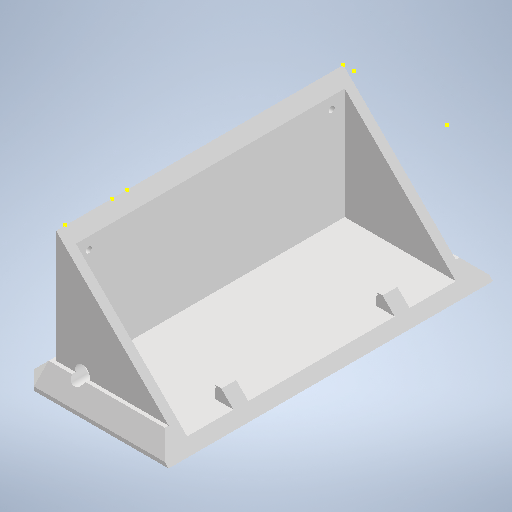
# Autodesk Inventor part: manuDisplayHolder
Saved by Autodesk Inventor 2025 (Build 290162000, 162)
## iProperties
Created: 2024-04-01
Part Number: manuDisplayHolder
Material: Generic
Document SubType Name: Modeling
Designer: 48791
Density: 1 g/cm^3
Appearance: Default
Author: 48791
Autodesk Inventor part; units mm, degrees
ref_plane "YZ Plane" through (0, 0, 0) normal (1, 0, 0) x (0, 1, 0)
ref_plane "XZ Plane" through (0, 0, 0) normal (0, 1, 0) x (-1, 0, 0)
sketch "Sketch1" plane through (0, 0, 0) normal (0, 0, 1) x (1, 0, 0)
  line L0 (0, 0) -> (0, -70.71)
  line L1 (0, -70.71) -> (70.71, -70.71)
  line L2 (70.71, -70.71) -> (0, 0)
  dimension "d0" = 70.71
  dimension "d1" = 70.71
  constraints: 6 end point, 1 perpendicular, 1 vertical
  measures "d0" distance of L0.start L0.end
  measures "d1" distance of L0.end L1.end
extrude "Extrusion1" add sketch "Sketch1" along normal blind 155
sketch "Sketch2" plane through (0, -70.71, 0) normal (0, -1, 0) x (1, 0, 0)
  point P0 (0, 0)
sketch "Sketch3" plane through (0, -70.71, 0) normal (0, -1, 0) x (1, 0, 0)
  point P0 (0, 0)
sketch "Sketch4" plane through (0, -70.71, 0) normal (0, -1, 0) x (1, 0, 0)
  point P0 (0, 0)
sketch "Sketch5" plane through (0, -70.71, 0) normal (0, -1, 0) x (1, 0, 0)
  line L0 (65.71, 150) -> (5.71, 150)
  line L1 (5.71, 150) -> (5.71, 5)
  line L2 (5.71, 5) -> (65.71, 5)
  line L3 (65.71, 5) -> (65.71, 150)
  line L4 (70.71, 0) -> (70.71, 155) projected
  line L5 (0, 0) -> (70.71, 0) projected
  dimension "d4" = 60
  dimension "d5" = 145
  dimension "d6" = 5
  dimension "d7" = 5
  constraints: 8 end point, 2 parallel, 1 horizontal, 1 perpendicular
  measures "d4" distance of L2.end L1.end
  measures "d5" distance of L1.end L0.end
  measures "d6" distance between parallel lines of L4 L3
  measures "d7" distance between parallel lines of L5 L2
extrude "Extrusion2" cut sketch "Sketch5" against normal blind 155
sketch "Sketch6" plane through (5.71, -70.71, 150) normal (1, 0, 0) x (0, 0, -1)
  line L0 (0, 0) -> (145, 0)
  line L1 (145, 0) -> (145, 5)
  line L2 (145, 5) -> (0, 5)
  line L3 (0, 5) -> (0, 0)
  point P0 (150, 70.71)
  dimension "d10" = 145
  dimension "d11" = 5
  constraints: 8 end point, 2 parallel, 1 horizontal, 1 perpendicular
  measures "d10" distance of L2.end L1.end
  measures "d11" distance of L1.end L0.end
extrude "Extrusion3" add sketch "Sketch6" along normal blind 60
sketch "Sketch7" plane through (5.71, -5.71, 150) normal (1, 0, 0) x (0, 0, -1)
  point P0 (150, 5.71)
sketch "Sketch8" plane through (65.71, -65.71, 150) normal (0, 0, -1) x (-1, 0, 0)
  point P0 (65.71, 65.71)
sketch "Sketch9" plane through (5.71, -65.71, 150) normal (0, 1, 0) x (1, 0, 0)
  point P0 (-5.71, 150)
sketch "Sketch10" plane through (5.71, -65.71, 150) normal (0, 1, 0) x (1, 0, 0)
  line L0 (60, 145) -> (60, 0) projected
  line L1 (60, 25) -> (50, 25)
  line L2 (50, 25) -> (50, 33)
  line L3 (50, 33) -> (60, 33)
  line L4 (60, 33) -> (60, 25)
  line L5 (60, 112) -> (50, 112)
  line L6 (50, 112) -> (50, 120)
  line L7 (50, 120) -> (60, 120)
  line L8 (60, 120) -> (60, 112)
  line L9 (60, 0) -> (0, 0) projected
  line L10 (0, 145) -> (60, 145) projected
  point P0 (-5.71, 150)
  point P1 (55, 25)
  point P2 (55, 120)
  point P3 (60, 33)
  dimension "d14" = 10
  dimension "d15" = 8
  dimension "d16" = 10
  dimension "d17" = 8
  dimension "d18" = 25
  dimension "d19" = 25
  constraints: 16 end point, 4 parallel, 2 horizontal, 2 midpoint, 2 perpendicular, 2 point on line
  measures "d14" distance of L2.end L3.end
  measures "d15" distance of L1.end L2.end
  measures "d16" distance of L6.end L7.end
  measures "d17" distance of L5.end L6.end
  measures "d18" distance from line of L9 point (55, 25)
  measures "d19" distance from line of L10 point (55, 120)
extrude "Extrusion4" add sketch "Sketch10" along normal blind 10
sketch "Sketch11" plane through (65.71, -65.71, 117) normal (0, 0, -1) x (-1, 0, 0)
  point P0 (65.71, 65.71)
sketch "Sketch12" plane through (65.71, -65.71, 117) normal (0, 0, -1) x (-1, 0, 0)
  line L0 (0, 10) -> (10, 10) projected
  line L1 (0, 0) -> (0, 10)
  line L2 (0, 10) -> (10, 10)
  line L3 (10, 10) -> (0, 0)
  point P0 (65.71, 65.71)
  constraints: 6 end point, 2 perpendicular
extrude "Extrusion5" cut sketch "Sketch12" against normal blind 15
sketch "Sketch13" plane through (65.71, -65.71, 30) normal (0, 0, -1) x (-1, 0, 0)
  line L0 (0, 0) -> (10, 0) projected
  line L1 (0, 0) -> (0, 10) projected
  line L2 (0, 0) -> (0, 10)
  line L3 (10, 0) -> (10, 10) projected
  line L4 (0, 10) -> (10, 10)
  line L5 (10, 10) -> (0, 0)
  point P0 (65.71, 65.71)
  constraints: 6 end point, 1 collinear, 1 perpendicular
extrude "Extrusion6" cut sketch "Sketch13" against normal blind 15 contours L1 L4 L5
sketch "Sketch14" plane through (65.71, -65.71, 150) normal (0, 0, -1) x (-1, 0, 0)
  circle A0 centre (51.4521, 6.4297) radius 4
  point P0 (65.71, 65.71)
  dimension "d26" = 8
  constraints: 1 centre point
  measures "d26" diameter of A0
extrude "Extrusion7" cut sketch "Sketch14" against normal blind 15
sketch "Sketch15" plane through (0, 0, 0) normal (0.7071068, 0.7071068, 0) x (-0.7071068, 0.7071068, 0)
  point P0 (0, 0)
sketch "Sketch16" plane through (0, 0, 0) normal (0.7071068, 0.7071068, 0) x (-0.7071068, 0.7071068, 0)
  point P0 (0, 0)
sketch "Sketch17" plane through (55.71, -65.71, 30) normal (-1, 0, 0) x (0, 0, 1)
  point P0 (-30, 65.71)
sketch "Sketch18" plane through (55.71, -65.71, 30) normal (-1, 0, 0) x (0, 0, 1)
  point P0 (-30, 65.71)
sketch "Sketch19" plane through (55.71, -65.71, 125) normal (0, 0, 1) x (1, 0, 0)
  point P0 (-55.71, 65.71)
sketch "Sketch20" plane through (55.71, -65.71, 125) normal (0, 0, 1) x (1, 0, 0)
  line L0 (-7.5736, 14.1421) -> (0.9117, 5.6569)
  line L1 (0.9117, 5.6569) -> (6.5685, 0)
  line L2 (6.5685, 0) -> (-0.5025, 0)
  line L3 (-0.5025, 0) -> (-2.6238, 2.1213)
  line L4 (-2.6238, 2.1213) -> (-4.0381, 3.5355)
  line L5 (-4.0381, 3.5355) -> (-2.2703, 5.3033)
  line L6 (-2.2703, 5.3033) -> (-9.3414, 12.3744)
  line L7 (-9.3414, 12.3744) -> (-7.5736, 14.1421)
  line L8 (0.9117, 5.6569) -> (-2.6238, 2.1213)
  line L9 (-46.4645, 45.9619) -> (-50, 49.4975)
  line L10 (-50, 49.4975) -> (-50, 56.5685)
  line L11 (-50, 56.5685) -> (-35.8579, 42.4264)
  line L12 (-35.8579, 42.4264) -> (-37.6256, 40.6586)
  line L13 (-37.6256, 40.6586) -> (-44.6967, 47.7297)
  line L14 (-44.6967, 47.7297) -> (-46.4645, 45.9619)
  point P0 (-55.71, 65.71)
  constraints: 30 end point, 1 horizontal, 1 vertical, 27 other
extrude "Extrusion8" cut sketch "Sketch20" against normal up to surface (95 mm away) contours L0 L8 L4 L5 L6 L7
sketch "Sketch21" plane through (0, -70.71, 0) normal (0, -1, 0) x (1, 0, 0)
  line L0 (0, 0) -> (70.71, 0) projected
  line L1 (70.71, 0) -> (70.71, 155) projected
  line L2 (0, 155) -> (70.71, 155) projected
  line L3 (0, 0) -> (0, 155) projected
  line L4 (-10, 165) -> (70.71, 165)
  line L5 (70.71, -10) -> (-10, -10)
  line L6 (-10, -10) -> (-10, 165)
  line L7 (0, 77.5) -> (70.71, 77.5)
  line L8 (35.355, 0) -> (35.355, 155)
  line L9 (70.71, 0) -> (70.71, 155) projected
  line L10 (70.71, -10) -> (70.71, 165)
  dimension "d31" = 10
  dimension "d32" = 10
  constraints: 12 end point, 4 midpoint, 2 point on line, 1 perpendicular, 1 other
  measures "d31" distance between parallel lines of L3 L6
  measures "d32" distance between parallel lines of L4 L2
extrude "Extrusion9" add sketch "Sketch21" against normal blind 10 contours L0 L10 L5 L6 L4 L2 L3
chamfer "Chamfer1" distance 8 angle 45 5 edges at (-10, -60.71, 77.5) (30.355, -60.71, 165) (-10, -65.71, 165) (30.355, -60.71, -10) (-10, -65.71, -10)
sketch "Sketch22" plane through (-2, -70.71, 165) normal (0, 0, 1) x (1, 0, 0)
  line L0 (72.71, 0) -> (62.71, 10) projected
  line L1 (72.71, 10) -> (62.71, 10) projected
  line L2 (72.71, 0) -> (72.71, 10) projected
  point P0 (2, 70.71)
extrude "Extrusion10" cut sketch "Sketch22" against normal blind 228.125
sketch "Sketch23" plane through (0, 0, 0) normal (-1, 0, 0) x (0, 0, 1)
  line L0 (36.1859, -20.6342) -> (112.0724, -20.6342) construction
  line L1 (112.0724, -20.6342) -> (112.0724, -41.0586) construction
  line L2 (112.0724, -41.0586) -> (36.1859, -41.0586) construction
  line L3 (36.1859, -41.0586) -> (36.1859, -20.6342) construction
  line L4 (0, -60.71) -> (155, -60.71) projected
  line L5 (155, 0) -> (155, -60.71) projected
  line L6 (0, 0) -> (155, 0) projected
  line L7 (0, 0) -> (0, -60.71) projected
  line L8 (0, 0) -> (155, 0) projected
  line L9 (74.1291, 0) -> (74.1291, -60.71) construction
  spline S0 degree 2 poles (50.979, -23.8756) (50.7548, -23.8756) (49.6859, -23.6859) (49.3928, -23.6859) knots 0 0 0 1 2 2 2
  spline S1 degree 2 poles (49.3928, -23.6859) (48.7893, -23.6859) (47.9617, -23.7204) knots 0 0 0 1 1 1
  line L10 (47.9617, -23.7204) -> (48.0307, -25.1859)
  spline S2 degree 2 poles (48.0307, -25.1859) (48.0307, -34.3928) (46.8066, -38.5825) knots 0 0 0 1 1 1
  spline S3 degree 2 poles (46.8066, -38.5825) (45.9962, -41.3583) (43.9445, -41.3583) knots 0 0 0 1 1 1
  spline S4 degree 2 poles (43.9445, -41.3583) (41.7893, -41.3583) (39.6859, -39.8066) knots 0 0 0 1 1 1
  spline S5 degree 2 poles (39.6859, -39.8066) (37.341, -38.0652) (37.341, -35.8238) knots 0 0 0 1 1 1
  spline S6 degree 2 poles (37.341, -35.8238) (37.341, -34.3066) (38.5997, -34.3066) knots 0 0 0 1 1 1
  spline S7 degree 2 poles (38.5997, -34.3066) (39.841, -34.3066) (39.841, -35.8066) knots 0 0 0 1 1 1
  spline S8 degree 2 poles (39.841, -35.8066) (39.841, -36.8238) (41.3066, -37.8411) knots 0 0 0 1 1 1
  spline S9 degree 2 poles (41.3066, -37.8411) (42.7031, -38.8066) (43.9445, -38.8066) knots 0 0 0 1 1 1
  spline S10 degree 2 poles (43.9445, -38.8066) (44.9617, -38.8066) (45.3583, -32.5825) knots 0 0 0 1 1 1
  spline S11 degree 2 poles (45.3583, -32.5825) (45.5479, -29.6514) (45.5479, -25.1859) knots 0 0 0 1 1 1
  spline S12 degree 2 poles (45.5479, -25.1859) (45.5479, -24.8411) (45.479, -23.8583) knots 0 0 0 1 1 1
  line L11 (45.479, -23.8583) -> (44.7376, -23.8756)
  spline S13 degree 2 poles (44.7376, -23.8756) (44.2548, -23.8756) (42.3066, -23.8066) (41.8238, -23.8066) knots 0 0 0 1 2 2 2
  spline S14 degree 2 poles (41.8238, -23.8066) (41.2721, -23.8066) (40.5307, -23.117) (40.5307, -22.5135) knots 0 0 0 1 2 2 2
  spline S15 degree 2 poles (40.5307, -22.5135) (40.5307, -21.2376) (42.2548, -21.2376) knots 0 0 0 1 1 1
  spline S16 degree 2 poles (42.2548, -21.2376) (42.6686, -21.2376) (44.3238, -21.3238) (44.7376, -21.3238) knots 0 0 0 1 2 2 2
  spline S17 degree 2 poles (44.7376, -21.3238) (45.5135, -21.3238) (48.6169, -21.1342) (49.3928, -21.1342) knots 0 0 0 1 2 2 2
  spline S18 degree 2 poles (49.3928, -21.1342) (52.2031, -21.1342) (52.2031, -22.5652) knots 0 0 0 1 1 1
  spline S19 degree 2 poles (52.2031, -22.5652) (52.2031, -23.0652) (51.8755, -23.4445) knots 0 0 0 1 1 1
  spline S20 degree 2 poles (51.8755, -23.4445) (51.5135, -23.8756) (50.979, -23.8756) knots 0 0 0 1 1 1
  spline S21 degree 2 poles (64.2893, -32.2894) (64.979, -32.7894) (65.9962, -33.8583) knots 0 0 0 1 1 1
  spline S22 degree 2 poles (65.9962, -33.8583) (67.1859, -35.0997) (68.0824, -35.8756) (68.0824, -36.3238) knots 0 0 0 1 2 2 2
  spline S23 degree 2 poles (68.0824, -36.3238) (68.0824, -36.7894) (67.41, -37.479) (66.979, -37.479) knots 0 0 0 1 2 2 2
  spline S24 degree 2 poles (66.979, -37.479) (66.6169, -37.479) (66.2721, -37.2204) knots 0 0 0 1 1 1
  spline S25 degree 2 poles (66.2721, -37.2204) (65.7893, -36.8583) (64.1686, -35.1687) knots 0 0 0 1 1 1
  spline S26 degree 2 poles (64.1686, -35.1687) (62.9272, -33.8756) (61.7721, -33.4273) knots 0 0 0 1 1 1
  spline S27 degree 2 poles (61.7721, -33.4273) (60.841, -33.0825) (60.841, -32.3928) knots 0 0 0 1 1 1
  spline S28 degree 2 poles (60.841, -32.3928) (60.841, -31.7721) (61.6859, -31.3756) knots 0 0 0 1 1 1
  spline S29 degree 2 poles (61.6859, -31.3756) (62.841, -30.8066) (64.2204, -29.3583) knots 0 0 0 1 1 1
  spline S30 degree 2 poles (64.2204, -29.3583) (66.1341, -27.3583) (66.8583, -26.7549) (67.2376, -26.7549) knots 0 0 0 1 2 2 2
  spline S31 degree 2 poles (67.2376, -26.7549) (67.6859, -26.7549) (68.3583, -27.4273) (68.3583, -27.8928) knots 0 0 0 1 2 2 2
  spline S32 degree 2 poles (68.3583, -27.8928) (68.3583, -28.3066) (67.979, -28.6859) knots 0 0 0 1 1 1
  spline S33 degree 2 poles (67.979, -28.6859) (66.8066, -29.9445) (64.2893, -32.2894) knots 0 0 0 1 1 1
  spline S34 degree 2 poles (77.7376, -40.4445) (75.8755, -40.4445) (74.3928, -39.6687) knots 0 0 0 1 1 1
  spline S35 degree 2 poles (74.3928, -39.6687) (72.7204, -38.7549) (72.1341, -37.1342) knots 0 0 0 1 1 1
  spline S36 degree 2 poles (72.1341, -37.1342) (72.0652, -36.9101) (72.0652, -36.7032) knots 0 0 0 1 1 1
  spline S37 degree 2 poles (72.0652, -36.7032) (72.0652, -36.2032) (72.8238, -35.548) (73.3238, -35.548) knots 0 0 0 1 2 2 2
  spline S38 degree 2 poles (73.3238, -35.548) (73.8066, -35.548) (74.1686, -35.9963) knots 0 0 0 1 1 1
  line L12 (74.1686, -35.9963) -> (74.7376, -36.8583)
  spline S39 degree 2 poles (74.7376, -36.8583) (75.1859, -37.4618) (76.6859, -38.0652) (77.7376, -38.0652) knots 0 0 0 1 2 2 2
  spline S40 degree 2 poles (77.7376, -38.0652) (79.0997, -38.0652) (80.1169, -37.2204) knots 0 0 0 1 1 1
  spline S41 degree 2 poles (80.1169, -37.2204) (81.1859, -36.3411) (81.1859, -35.048) knots 0 0 0 1 1 1
  spline S42 degree 2 poles (81.1859, -35.048) (81.1859, -33.1859) (79.8066, -32.0652) knots 0 0 0 1 1 1
  spline S43 degree 2 poles (79.8066, -32.0652) (78.5997, -31.0997) (76.5997, -30.8928) knots 0 0 0 1 1 1
  spline S44 degree 2 poles (76.5997, -30.8928) (75.2204, -30.7549) (75.2204, -29.7721) knots 0 0 0 1 1 1
  spline S45 degree 2 poles (75.2204, -29.7721) (75.2204, -29.048) (76.2893, -28.6687) knots 0 0 0 1 1 1
  line L13 (76.2893, -28.6687) -> (79.2548, -27.9445)
  spline S46 degree 2 poles (79.2548, -27.9445) (80.0997, -27.6342) (80.9617, -26.5825) (80.979, -25.8238) knots 0 0 0 1 2 2 2
  spline S47 degree 2 poles (80.979, -25.8238) (80.9962, -24.7376) (80.1341, -24.0652) knots 0 0 0 1 1 1
  spline S48 degree 2 poles (80.1341, -24.0652) (79.2376, -23.3756) (77.5997, -23.3756) knots 0 0 0 1 1 1
  spline S49 degree 2 poles (77.5997, -23.3756) (76.7548, -23.3756) (75.979, -23.7894) knots 0 0 0 1 1 1
  line L14 (75.979, -23.7894) -> (74.5824, -24.6687)
  spline S50 degree 2 poles (74.5824, -24.6687) (74.1686, -24.9273) (73.9272, -24.9273) knots 0 0 0 1 1 1
  spline S51 degree 2 poles (73.9272, -24.9273) (73.4272, -24.9273) (72.7204, -24.1687) (72.7204, -23.6859) knots 0 0 0 1 2 2 2
  spline S52 degree 2 poles (72.7204, -23.6859) (72.7204, -22.7032) (74.6169, -21.8066) knots 0 0 0 1 1 1
  spline S53 degree 2 poles (74.6169, -21.8066) (76.2548, -20.9963) (77.3238, -20.9963) knots 0 0 0 1 1 1
  spline S54 degree 2 poles (77.3238, -20.9963) (79.979, -20.9963) (81.5307, -22.1687) knots 0 0 0 1 1 1
  spline S55 degree 2 poles (81.5307, -22.1687) (83.2031, -23.4273) (83.2031, -25.7721) knots 0 0 0 1 1 1
  spline S56 degree 2 poles (83.2031, -25.7721) (83.2031, -28.6859) (80.8583, -29.5997) knots 0 0 0 1 1 1
  spline S57 degree 2 poles (80.8583, -29.5997) (80.6514, -29.6859) (80.3755, -29.7721) knots 0 0 0 1 1 1
  spline S58 degree 2 poles (80.3755, -29.7721) (82.0135, -30.3928) (83.6514, -32.8066) (83.6514, -34.5997) knots 0 0 0 1 2 2 2
  spline S59 degree 2 poles (83.6514, -34.5997) (83.6514, -37.048) (80.2204, -40.4445) (77.7376, -40.4445) knots 0 0 0 1 2 2 2
  spline S60 degree 2 poles (106.5997, -39.7894) (104.6859, -41.0997) (101.0824, -41.0997) knots 0 0 0 1 1 1
  spline S61 degree 2 poles (101.0824, -41.0997) (100.1859, -41.0997) (99.0307, -40.8066) knots 0 0 0 1 1 1
  spline S62 degree 2 poles (99.0307, -40.8066) (97.6341, -40.479) (96.9272, -39.9445) knots 0 0 0 1 1 1
  line L15 (96.9272, -39.9445) -> (96.7893, -39.9445)
  spline S63 degree 2 poles (96.7893, -39.9445) (96.2721, -39.9445) (95.5479, -39.2032) (95.5479, -38.6687) knots 0 0 0 1 2 2 2
  spline S64 degree 2 poles (95.5479, -38.6687) (95.5479, -37.3756) (95.7893, -32.2032) (95.7893, -30.8928) knots 0 0 0 1 2 2 2
  spline S65 degree 2 poles (95.7893, -30.8928) (95.7893, -29.4445) (95.6686, -23.7032) (95.6686, -22.2549) knots 0 0 0 1 2 2 2
  spline S66 degree 2 poles (95.6686, -22.2549) (95.6686, -21.7549) (96.7031, -20.6342) (97.2204, -20.6342) knots 0 0 0 1 2 2 2
  spline S67 degree 2 poles (97.2204, -20.6342) (97.5307, -20.6342) (99.2031, -21.4618) knots 0 0 0 1 1 1
  spline S68 degree 2 poles (99.2031, -21.4618) (101.1169, -22.3928) (101.41, -22.4963) knots 0 0 0 1 1 1
  spline S69 degree 2 poles (101.41, -22.4963) (104.9272, -23.6859) (107.3928, -26.1687) knots 0 0 0 1 1 1
  spline S70 degree 2 poles (107.3928, -26.1687) (110.3066, -29.0997) (110.3066, -32.617) knots 0 0 0 1 1 1
  spline S71 degree 2 poles (110.3066, -32.617) (110.3066, -34.7376) (108.3066, -38.617) (106.5997, -39.7894) knots 0 0 0 1 2 2 2
  spline S72 degree 2 poles (103.9962, -26.7032) (102.7376, -25.8756) (98.1686, -23.8583) knots 0 0 0 1 1 1
  line L16 (98.1686, -23.8583) -> (98.2376, -27.4273)
  line L17 (98.2376, -27.4273) -> (98.2721, -30.979)
  line L18 (98.2721, -30.979) -> (98.0824, -37.7204)
  spline S73 degree 2 poles (98.0824, -37.7204) (98.1686, -37.7549) (98.341, -37.8928) knots 0 0 0 1 1 1
  spline S74 degree 2 poles (98.341, -37.8928) (99.4272, -38.617) (101.0824, -38.617) knots 0 0 0 1 1 1
  spline S75 degree 2 poles (101.0824, -38.617) (103.91, -38.617) (105.1859, -37.7549) knots 0 0 0 1 1 1
  spline S76 degree 2 poles (105.1859, -37.7549) (106.3928, -36.9273) (107.8066, -34.1687) (107.8066, -32.6859) knots 0 0 0 1 2 2 2
  spline S77 degree 2 poles (107.8066, -32.6859) (107.8066, -29.1859) (103.9962, -26.7032) knots 0 0 0 1 1 1
  constraints: 2 end point, 2 point on line, 1 perpendicular, 2 other
extrude "Extrusion11" cut sketch "Sketch23" against normal blind 1 contours S0 S1 L10 S2 S3 S4 S5 S6 S7 S8 S9 S10 S11 S12 L11 S13 S14 S15 S16 S17 S18 S19 S20 | S21 S22 S23 S24 S25 S26 S27 S28 S29 S30 S31 S32 S33 | S34 S35 S36 S37 S38 L12 S39 S40 S41 S42 S43 S44 S45 L13 S46 S47 S48 S49 L14 S50 S51 S52 S53 S54 S55 S56 S57 S58 S59 | S60 S61 S62 L15 S63 S64 S65 S66 S67 S68 S69 S70 S71
sketch "Sketch24" plane through (0, 0, 0) normal (-1, 0, 0) x (0, 0, 1)
  circle A0 centre (12, -12) radius 1.6
  line L0 (0, 0) -> (155, 0) projected
  line L1 (0, 0) -> (0, -60.71) projected
  line L2 (0, 0) -> (12, 0)
  line L3 (12, 0) -> (12, -12)
  line L4 (12, -12) -> (0, -12)
  line L5 (0, -12) -> (0, 0)
  line L6 (77.5, 0) -> (77.5, -60.71) construction
  line L7 (0, -60.71) -> (155, -60.71) projected
  circle A1 centre (143, -12) radius 1.6
  dimension "d42" = 3.2
  dimension "d47" = 12
  dimension "d48" = 12
  constraints: 10 end point, 2 centre point, 2 midpoint, 2 parallel, 1 coincident, 1 horizontal, 1 perpendicular, 1 symmetric about line, 1 other
  measures "d42" diameter of A0
  measures "d47" distance between parallel lines of L1 L3
  measures "d48" distance of L2.end L3.end
ref_plane "Work Plane1" through (33.9943, -34.1764, 5) normal (0.7071068, 0.7071068, 0) x (0, 0, 1)
extrude "Extrusion12" cut sketch "Sketch24" along normal up to surface contours A0 L4 L3 | L3 L4 A0 | A1 surface through (33.9943, -34.1764, 5) normal (0.7071068, 0.7071068, 0)
sketch "Sketch25" plane through (14.2579, -59.2803, 155) normal (0, 0, -1) x (-1, 0, 0)
  arc A0 (-3.7358, -1.4297) -> (3.7358, -1.4297) centre (0, 0) ccw projected
  line L0 (-3.7358, -1.4297) -> (3.7358, -1.4297) projected
  point P0 (14.2579, 59.2803)
extrude "Extrusion13" cut sketch "Sketch25" against normal blind 21.75
sketch "Sketch26" plane through (55.71, -55.71, 30) normal (-1, 0, 0) x (0, 0, 1)
  line L0 (87, 0) -> (95, 0) projected
  line L1 (87, -3.4315) -> (95, -3.4315) projected
  line L2 (95, -3.4315) -> (95, 0) projected
  line L3 (87, 0) -> (95, 0) projected
  line L4 (87, -3.4315) -> (87, 0) projected
  line L5 (0, -3.4315) -> (8, -3.4315) projected
  line L6 (8, -3.4315) -> (8, 0) projected
  line L7 (0, 0) -> (8, 0) projected
  line L8 (0, -3.4315) -> (0, 0) projected
  point P0 (-30, 55.71)
extrude "Extrusion14" cut sketch "Sketch26" against normal blind 21.75
body "Solid1"
